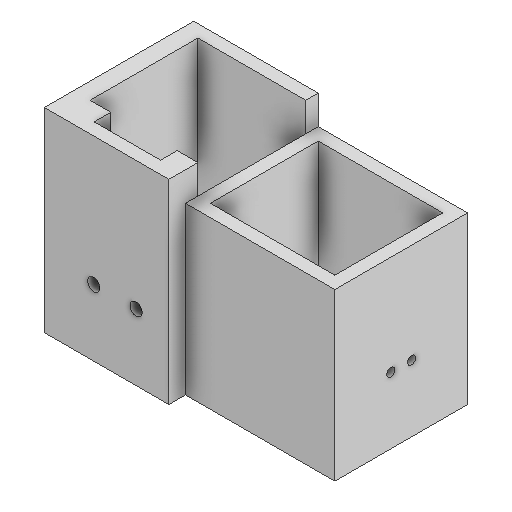
# Autodesk Inventor part: Base
Saved by Autodesk Inventor 2027 (Build 310192060, 192F)
## iProperties
Created: 2023-05-04
Part Number: Base
Material: Genérico
Document SubType Name: Modeling
Designer: barof
Density: 1 g/cm^3
Appearance: Padrão
Author: barof
## iProperties of the stored document Base_3DPrint.ipt
Created: 2023-05-04
Part Number: Base_3DPrint
Material: Genérico
Document SubType Name: Modeling
Designer: barof
Density: 1 g/cm^3
Appearance: Padrão
Author: barof
Autodesk Inventor part; units mm, degrees
ref_plane "YZ Plane" through (0, 0, 0) normal (1, 0, 0) x (0, 1, 0)
ref_plane "XZ Plane" through (0, 0, 0) normal (0, 1, 0) x (-1, 0, 0)
ref_plane "XY Plane" through (0, 0, 0) normal (0, 0, 1) x (1, 0, 0)
sketch "Esboço1" plane through (0, 0, 0) normal (0, 1, 0) x (-1, 0, 0)
  line L0 (0, 0) -> (0, -16)
  line L1 (0, -16) -> (-34.5, -16)
  line L2 (-34.5, -16) -> (-34.5, 0)
  line L3 (-34.5, 0) -> (0, 0)
  line L4 (-3.5, -14.5) -> (-16.5, -14.5)
  line L5 (-16.5, -14.5) -> (-16.5, -1.5)
  line L6 (-16.5, -1.5) -> (-3.5, -1.5)
  line L7 (-18, -14.5) -> (-33, -14.5)
  line L8 (-33, -14.5) -> (-33, -1.5)
  line L9 (-33, -1.5) -> (-18, -1.5)
  line L10 (-18, -1.5) -> (-18, -14.5)
  line L11 (-3.5, -14.5) -> (-3.5, -12)
  line L12 (-3.5, -12) -> (-1.5, -12)
  line L13 (-1.5, -12) -> (-1.5, -4)
  line L14 (-1.5, -4) -> (-3.5, -4)
  line L15 (-3.5, -4) -> (-3.5, -1.5)
  point P0 (-34.5, -8)
  dimension "d0" = 13
  dimension "d1" = 13
  dimension "d2" = 15
  dimension "d3" = 13
  dimension "d4" = 8
  dimension "d5" = 2.5
  dimension "d6" = 1.5
  dimension "d7" = 1.5
  dimension "d8" = 2
  dimension "d9" = 1.5
  dimension "d10" = 1.5
  dimension "d11" = 1.5
  constraints: 32 end point, 9 perpendicular, 3 parallel, 2 horizontal, 2 point on line, 2 vertical, 1 midpoint
  measures "d0" distance of L4.start L4.end
  measures "d1" distance of L4.end L5.end
  measures "d2" distance of L7.start L7.end
  measures "d3" distance of L7.end L8.end
  measures "d4" distance of L12.end L13.end
  measures "d5" distance of L4.start L11.end
  measures "d6" distance between parallel lines of L6 L3
  measures "d7" distance between parallel lines of L0 L13
  measures "d8" distance of L13.end L14.end
  measures "d9" distance between parallel lines of L10 L5
  measures "d10" distance between parallel lines of L2 L8
  measures "d11" distance between parallel lines of L1 L7
extrude "Extrusão1" add sketch "Esboço1" along normal blind 1.5 contours L4 L5 L6 L15 L14 L13 L12 L11 | L7 L8 L9 L10
extrude "Extrusão2" add sketch "Esboço1" along normal blind 20
sketch "Esboço2" plane through (0, 0, -16) normal (-1, 0, 0) x (0, 0, 1)
  line L0 (12, 20) -> (4, 20) projected
  line L1 (8, 20) -> (8, 0)
  line L2 (0, 0) -> (0, 20) projected
  circle A0 centre (5.45, 8) radius 0.5
  circle A1 centre (10.55, 8) radius 0.5
  line L3 (0, 0) -> (16, 0) projected
  dimension "d23" = 8
  constraints: 2 centre point, 2 end point, 1 midpoint, 1 vertical
  measures "d23" distance from line of L3 A1.centre
extrude "Extrusão3" cut sketch "Esboço2" against normal blind 10
sketch "Esboço3" plane through (34.5, 0, 0) normal (1, 0, 0) x (0, 0, -1)
  line L0 (0, 20) -> (16, 20) projected
  line L1 (8, 20) -> (8, 0)
  circle A0 centre (6.75, 8) radius 0.5
  circle A1 centre (9.25, 8) radius 0.5
  line L2 (0, 0) -> (16, 0) projected
  line L3 (11, 16) -> (11, 8)
  line L4 (11, 8) -> (5, 8)
  line L5 (5, 8) -> (5, 16)
  circle A2 centre (5, 12) radius 1.5
  circle A3 centre (11, 12) radius 1.5
  dimension "d26" = 1
  dimension "d27" = 1
  dimension "d28" = 8
  dimension "d29" = 8
  dimension "d30" = 1.25
  dimension "d31" = 1.25
  dimension "d78" = 3
  dimension "d79" = 3
  dimension "d80" = 3
  dimension "d81" = 3
  constraints: 8 end point, 4 centre point, 3 midpoint, 1 parallel, 1 vertical
  measures "d26" diameter of A0
  measures "d27" diameter of A1
  measures "d28" distance from line of L2 A0.centre
  measures "d29" distance from line of L2 A1.centre
  measures "d30" distance from line of L1 A0.centre
  measures "d31" distance from line of L1 A1.centre
  measures "d78" diameter of A2
  measures "d79" diameter of A3
  measures "d80" distance between parallel lines of L1 L3
  measures "d81" distance between parallel lines of L1 L5
extrude "Extrusão4" cut sketch "Esboço3" against normal blind 10 contours L4 A0 | A1 L4 | L4 A1 | A0 L4
sketch "Esboço4" plane through (18, 1.5, -14.5) normal (1, 0, 0) x (0, 0, -1)
  line L0 (-14.5, -1.5) -> (1.5, -1.5) projected
  line L1 (-6.5, -1.5) -> (-6.5, 18.5)
  line L2 (0, 18.5) -> (-13, 18.5) projected
  circle A0 centre (-6.5, 6.5) radius 2.5
  line L3 (0, 0) -> (-13, 0) projected
  dimension "d40" = 5
  dimension "d42" = 6.5
  constraints: 2 end point, 2 midpoint, 1 centre point, 1 point on line
  measures "d40" diameter of A0
  measures "d42" distance from line of A0.centre L3
extrude "Extrusão5" cut sketch "Esboço4" against normal blind 10
sketch "Esboço6" plane through (0, 20, 0) normal (0, 1, 0) x (1, 0, 0)
  line L0 (0, 0) -> (34.5, 0) projected
  line L1 (0, 0) -> (16.5, 0)
  line L2 (0, 0) -> (16.5, 0) construction
  line L3 (16.5, 14.5) -> (16.5, 1.5) projected
  line L4 (16.5, 0) -> (16.5, 1.5)
  line L5 (16.5, 1.5) -> (3.5, 1.5) projected
  line L6 (16.5, 1.5) -> (3.5, 1.5)
  line L7 (3.5, 1.5) -> (3.5, 4) projected
  line L8 (3.5, 1.5) -> (3.5, 4)
  line L9 (3.5, 4) -> (1.5, 4) projected
  line L10 (3.5, 4) -> (1.5, 4)
  line L11 (1.5, 4) -> (1.5, 12)
  line L12 (1.5, 12) -> (3.5, 12) projected
  line L13 (1.5, 12) -> (3.5, 12)
  line L14 (3.5, 12) -> (3.5, 14.5) projected
  line L15 (3.5, 12) -> (3.5, 14.5)
  line L16 (3.5, 14.5) -> (16.5, 14.5) projected
  line L17 (3.5, 14.5) -> (16.5, 14.5)
  line L18 (16.5, 14.5) -> (16.5, 16)
  line L19 (34.5, 16) -> (0, 16) projected
  line L20 (0, 16) -> (0, 0) projected
  line L21 (0, 16.0004) -> (0, 0)
  dimension "d66" = 16.5
  dimension "d67" = 0
  constraints: 24 end point, 8 collinear, 2 point on line, 1 horizontal, 1 perpendicular
  measures "d66" distance of L0.start L1.end
  measures "d67" distance between parallel lines of L2 L1
extrude "Extrusão8" add sketch "Esboço6" along normal blind 3.5 contours L20 L19 L18 L16 L14 L12 L11 L9 L7 L5 L4 L0
sketch "Sketch8" plane through (0, 23.5, 0) normal (0, 1, 0) x (1, 0, 0)
  line L0 (3.5, 1.5) -> (16.5, 1.5) projected
  line L1 (6, 1.5) -> (6, -0.5)
  line L2 (6, -0.5) -> (14, -0.5)
  line L3 (14, -0.5) -> (14, 1.5)
  line L4 (16.5, 1.5) -> (14, 1.5)
  line L5 (3.5, 1.5) -> (3.5, -2)
  line L6 (3.5, -2) -> (16.5, -2)
  line L7 (16.5, -2) -> (16.5, 1.5)
  line L8 (0, 0) -> (34.5, 0) projected
  point P0 (6, 0)
  point P1 (14, 0)
  dimension "d86" = 8
  dimension "d87" = 2.5
  dimension "d88" = 2
  dimension "d89" = 2
  dimension "d90" = 3.5
  constraints: 14 end point, 3 perpendicular, 2 point on line, 2 vertical, 1 collinear
  measures "d86" distance of L1.end L2.end
  measures "d87" distance from line of L0.start L1
  measures "d88" distance of L2.end L3.end
  measures "d89" distance of L1.start L1.end
  measures "d90" distance of L0.start L5.end
extrude "Extrusion12" add sketch "Sketch8" against normal up to surface (23.5 mm away) contours L0 L1 L8 L5 | L8 L1 L2 L3 L7 L6 L5 | L0 L7 L8 L3
extrude "Extrusion13" cut sketch "Sketch8" against normal blind 22 contours L0 L3 L8 L1
sketch "Sketch9" plane through (0, 23.5, 0) normal (0, 1, 0) x (1, 0, 0)
  line L0 (34.5, 16) -> (0, 16) projected
  line L1 (0, 0) -> (3.5, 0) projected
  line L2 (0, 16) -> (1.5, 16)
  line L3 (1.5, 16) -> (1.5, 0)
  line L4 (1.5, 0) -> (0, 0)
  line L5 (0, 0) -> (0, 16)
  line L6 (3.5, 12) -> (1.5, 12) projected
  line L7 (3.5, 1.5) -> (3.5, 4) projected
  line L8 (3.5, 12) -> (3.5, 4)
  dimension "d95" = 1.5
  constraints: 10 end point, 2 parallel, 1 collinear, 1 horizontal, 1 perpendicular, 1 point on line
  measures "d95" distance of L3.end L4.end
extrude "Extrusion14" cut sketch "Sketch9" against normal through all
sketch "Sketch10" plane through (0, 23.5, 0) normal (0, 1, 0) x (1, 0, 0)
  line L0 (3.5, 14.5) -> (3.5, 12) projected
  line L1 (1.5, 12) -> (1.5, 4) projected
  line L2 (3.5, 12) -> (1.5, 12)
  line L3 (1.5, 12) -> (1.5, 4)
  line L4 (1.5, 4) -> (3.5, 4)
  line L5 (3.5, 4) -> (3.5, 12)
  point P0 (0, 0)
  constraints: 8 end point, 2 parallel, 1 horizontal, 1 perpendicular
extrude "Extrusion15" add sketch "Sketch10" against normal up to surface (22 mm away)
sketch "Sketch11" plane through (0, 0, 0) normal (0, -1, 0) x (1, 0, 0)
  line L0 (6, 0) -> (14, 0) projected
  line L1 (6, 0.5) -> (14, 0.5) projected
  line L2 (6, 0) -> (14, 0)
  line L3 (14, 0) -> (14, 0.5)
  line L4 (14, 0.5) -> (6, 0.5)
  line L5 (6, 0.5) -> (6, 0)
  point P0 (0, 0)
  constraints: 8 end point, 2 parallel, 1 horizontal, 1 perpendicular
extrude "Extrusion16" add sketch "Sketch11" against normal blind 1.5
sketch "Sketch12" plane through (0, 23.5, 0) normal (0, 1, 0) x (1, 0, 0)
  line L0 (1.5, 16) -> (1.5, 0) projected
  line L1 (3.5, -2) -> (3.5, 0) projected
  line L2 (1.5, 0) -> (3.5, 0)
  line L3 (3.5, 0) -> (3.5, -2)
  line L4 (3.5, -2) -> (1.5, -2)
  line L5 (1.5, -2) -> (1.5, 0)
  point P0 (0, 0)
  constraints: 8 end point, 2 parallel, 1 horizontal, 1 perpendicular
extrude "Extrusion17" add sketch "Sketch12" against normal up to surface (23.5 mm away)
sketch "Sketch13" plane through (16.5, 0, 2) normal (0, 0, 1) x (1, 0, 0)
  line L0 (-13, 23.5) -> (0, 23.5) projected
  line L1 (-6.5, 23.5) -> (-6.5, 0)
  circle A0 centre (-3.95, 8) radius 0.75
  circle A1 centre (-9.05, 8) radius 0.75
  line L2 (0, 0) -> (-15, 0) projected
  line L3 (0, 23.5) -> (0, 0) projected
  point P0 (-16.5, 0)
  dimension "d104" = 1.5
  dimension "d105" = 1.5
  dimension "d106" = 8
  dimension "d107" = 8
  dimension "d108" = 6.5
  dimension "d109" = 2.55
  dimension "d110" = 2.55
  constraints: 2 centre point, 2 end point, 1 midpoint, 1 vertical
  measures "d104" diameter of A0
  measures "d105" diameter of A1
  measures "d106" distance from line of L2 A1.centre
  measures "d107" distance from line of L2 A0.centre
  measures "d108" distance between parallel lines of L3 L1
  measures "d109" distance from line of L1 A1.centre
  measures "d110" distance from line of A0.centre L1
extrude "Extrusion18" cut sketch "Sketch13" against normal blind 10 contours A0 | A1
